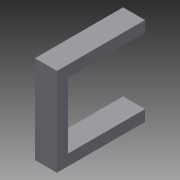
# Autodesk Inventor part: Camera Mount
Saved by Autodesk Inventor 2014 (Build 180170000, 170)
## iProperties
Created: 2014-01-20
Part Number: Camera Mount
Material: Generic
Document SubType Name: Modeling
Designer: Andrew Toennies
Density: 1 g/cm^3
Appearance: Default
Author: Andrew Toennies
Autodesk Inventor part; units mm, degrees
ref_plane "YZ Plane" through (0, 0, 0) normal (1, 0, 0) x (0, 1, 0)
ref_plane "XZ Plane" through (0, 0, 0) normal (0, 1, 0) x (-1, 0, 0)
ref_plane "XY Plane" through (0, 0, 0) normal (0, 0, 1) x (1, 0, 0)
sketch "Sketch1" plane through (0, 0, 0) normal (1, 0, 0) x (0, 1, 0)
  line L0 (0, 0) -> (0, -50.8)
  line L1 (0, -50.8) -> (6.35, -50.8)
  line L2 (6.35, -50.8) -> (6.35, -6.35)
  line L3 (6.35, -6.35) -> (44.45, -6.35)
  line L4 (44.45, -6.35) -> (44.45, -50.8)
  line L5 (44.45, -50.8) -> (50.8, -50.8)
  line L6 (50.8, -50.8) -> (50.8, 0)
  line L7 (50.8, 0) -> (0, 0)
  dimension "d0" = 50.8
  dimension "d1" = 6.35
  dimension "d2" = 44.45
  dimension "d3" = 38.1
  dimension "d4" = 44.45
  dimension "d5" = 6.35
  constraints: 16 end point, 5 parallel, 1 collinear, 1 perpendicular, 1 vertical
  measures "d0" distance of L0.start L0.end
  measures "d1" distance of L0.end L1.end
  measures "d2" distance of L1.end L2.end
  measures "d3" distance of L2.end L3.end
  measures "d4" distance of L3.end L4.end
  measures "d5" distance of L4.end L5.end
extrude "Extrusion1" add sketch "Sketch1" along normal blind 12.7
body "Solid1"
